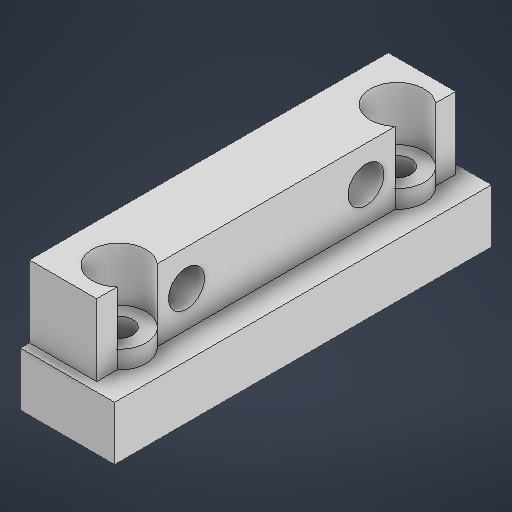
# Autodesk Inventor part: Z Axis Stepper Bracket
Saved by Autodesk Inventor 2025.1 (Build 291241000, 241)
## iProperties
Created: 2025-01-21
Part Number: Z Axis Stepper Bracket
Material: Generic
Document SubType Name: Modeling
Designer: jerem
Density: 1 g/cm^3
Appearance: Default
Author: jerem
Autodesk Inventor part; units mm, degrees
ref_plane "YZ Plane" through (0, 0, 0) normal (1, 0, 0) x (0, 1, 0)
ref_plane "XZ Plane" through (0, 0, 0) normal (0, 1, 0) x (-1, 0, 0)
ref_plane "XY Plane" through (0, 0, 0) normal (0, 0, 1) x (1, 0, 0)
sketch "Sketch1" plane through (0, 0, 0) normal (0, 1, 0) x (-1, 0, 0)
  line L0 (-4.5, -21) -> (4.5, -21)
  line L1 (4.5, -21) -> (4.5, 21) construction
  line L2 (4.5, 21) -> (-4.5, 21)
  line L3 (-4.5, 21) -> (-4.5, -21)
  line L4 (-4.5, -21) -> (4.5, 21) construction
  line L5 (4.5, -21) -> (-4.5, 21) construction
  circle A0 centre (0.5, 15.5) radius 1.5
  circle A1 centre (0.5, -15.5) radius 1.5
  line L6 (0.5, 15.5) -> (0.5, -15.5) construction
  line L7 (4.5, 0) -> (0.5, 0) construction
  line L8 (6, 20) -> (-1.5, 20)
  line L9 (-1.5, 20) -> (-1.5, -20)
  line L10 (-1.5, -20) -> (6, -20)
  circle A2 centre (0.5, 15.5) radius 3
  circle A3 centre (0.5, -15.5) radius 3
  line L11 (4.5, -21) -> (6, -21)
  line L12 (6, -21) -> (6, 21)
  line L13 (6, 21) -> (4.5, 21)
  point P0 (0, 0)
  point P1 (-1.5, 0)
  point P2 (-1.5, 17.7361)
  point P3 (-1.5, 13.2639)
  point P4 (-1.5, -13.2639)
  point P5 (-1.5, -17.7361)
  dimension "d0" = 42
  dimension "d1" = 9
  dimension "d2" = 3
  dimension "d3" = 4
  dimension "d4" = 31
  dimension "d7" = 40
  dimension "d8" = 6
  dimension "d18" = 1.5
  dimension "d19" = 1.5
  dimension "d24" = 1.5
  constraints: 28 end point, 6 perpendicular, 5 midpoint, 4 centre point, 3 horizontal, 3 point on line, 2 coincident, 2 parallel, 2 vertical, 1 collinear, 1 equal radius
  measures "d0" distance between parallel lines of L0 L2
  measures "d1" distance between parallel lines of L1 L3
  measures "d2" diameter of A0
  measures "d3" distance between parallel lines of L1 L6
  measures "d4" distance of L6.end L6.start
  measures "d7" distance between parallel lines of L10 L8
  measures "d8" distance between parallel lines of L9 L1
  measures "d18" radial gap between concentric circles of A1 A3
  measures "d19" radial gap between concentric circles of A2 A0
  measures "d24" distance between parallel lines of L1 L12
extrude "Extrusion1" add sketch "Sketch1" along normal blind 6
extrude "Extrusion2" add sketch "Sketch1" along normal blind 8 from surface at 6 contours L10 L9 A3 A2 L8 L12
sketch "Sketch3" plane through (1.5, 6, 20) normal (1, 0, 0) x (0, 0, -1)
  line L0 (2.2639, 8) -> (0, 8) projected
  line L1 (0, 0) -> (0, 8) projected
  line L2 (40, 0) -> (37.7361, 0) projected
  line L3 (40, 0) -> (40, 8) projected
  line L4 (10, 4) -> (30, 4) construction
  line L5 (37, 0) -> (37, -6) construction
  line L6 (20, 4) -> (20, 8) construction
  line L7 (40, 8) -> (0, 8) construction
  circle A0 centre (10, 4) radius 2
  circle A1 centre (30, 4) radius 2
  circle A2 centre (10, 4) radius 4
  circle A3 centre (30, 4) radius 4
  line L8 (40, 8) -> (37.7361, 8) projected
  line L9 (37.7361, 0) -> (37.7361, 8) projected
  line L10 (2.2639, 0) -> (0, 0) projected
  line L11 (2.2639, 0) -> (2.2639, 8) projected
  line L12 (33.2639, 8) -> (6.7361, 8) projected
  line L13 (6.7361, 0) -> (6.7361, 8) projected
  line L14 (33.2639, 0) -> (6.7361, 0) projected
  line L15 (33.2639, 0) -> (33.2639, 8) projected
  point P0 (20, -6)
  dimension "d11" = 20
  dimension "d12" = 4
  dimension "d15" = 4
  dimension "d22" = 8
  constraints: 4 centre point, 4 coincident, 4 end point, 2 equal radius, 2 midpoint, 1 perpendicular, 1 vertical, 2 other
  measures "d11" distance of L4.start L4.end
  measures "d12" diameter of A0
  measures "d15" distance between parallel lines of L2 L4
  measures "d22" diameter of A2
extrude "Extrusion4" add sketch "Sketch1" along normal blind 8 from surface at 0 contours A3 L9 | L9 A3 | A2 L9 | L9 A2
extrude "Extrusion3" cut sketch "Sketch3" against normal through all contours A0 | A1
equation "\"d18\" = d19"
body "Solid1"
